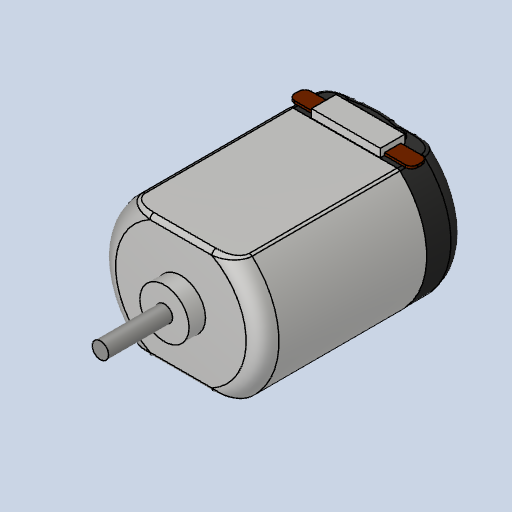
# Autodesk Inventor part: 3V DC Electromotor
Saved by Autodesk Inventor 2023 (Build 270158000, 158)
## iProperties
Created: 2020-10-25
Part Number: 3V DC Electromotor
Material: Aluminum 6061
Document SubType Name: Modeling
Designer: Niels
Density: 2.7 g/cm^3
Appearance: Aluminum - Flat
MAAT: ØLxBxD
Author: Niels
Autodesk Inventor part; units mm, degrees
ref_plane "YZ Plane" through (0, 0, 0) normal (1, 0, 0) x (0, 1, 0)
ref_plane "XZ Plane" through (0, 0, 0) normal (0, 1, 0) x (-1, 0, 0)
ref_plane "XY Plane" through (0, 0, 0) normal (0, 0, 1) x (1, 0, 0)
sketch "Sketch1" plane through (0, 0, 0) normal (0, 0, 1) x (1, 0, 0)
  circle A0 centre (0, 0) radius 9.95
  line L0 (-6.53854, 7.5) -> (6.53854, 7.5)
  line L1 (6.53854, -7.5) -> (-6.53854, -7.5)
  dimension "d0" = 19.9
  dimension "d2" = 15
  constraints: 4 end point, 4 point on circle, 1 centre point, 1 coincident, 1 horizontal, 1 parallel, 1 vertical alignment
  measures "d0" diameter of A0
  measures "d2" distance between parallel lines of L1 L0
extrude "Extrusion1" add sketch "Sketch1" along normal blind 20 contours A0 L1 L0
sketch "Sketch2" plane through (0, 0, 0) normal (0, 0, -1) x (-1, 0, 0)
  arc A0 (6.53854, -7.5) -> (6.53854, 7.5) centre (0, 0) ccw
  line L0 (-6.53854, 7.5) -> (6.53854, 7.5)
  arc A1 (-6.53854, 7.5) -> (-6.53854, -7.5) centre (0, 0) ccw
  line L1 (6.53854, -7.5) -> (-6.53854, -7.5)
  arc A2 (6.519778, -7.45) -> (6.519778, 7.45) centre (0, 0) ccw
  line L2 (6.519778, -7.45) -> (-6.519778, -7.45)
  arc A3 (-6.519778, 7.45) -> (-6.519778, -7.45) centre (0, 0) ccw
  line L3 (-6.519778, 7.45) -> (6.519778, 7.45)
  dimension "d5" = 0.05
  constraints: 4 end point, 4 point on circle, 2 centre point, 3 other
  measures "d5" distance between parallel lines of L0 L3
extrude "Extrusion2" add sketch "Sketch2" along normal blind 5 contours L2 A3 L3 A2
sketch "Sketch3" plane through (0, 0, 20) normal (0, 0, 1) x (1, 0, 0)
  circle A0 centre (0, 0) radius 3
  dimension "d8" = 6
  constraints: 1 centre point, 1 coincident
  measures "d8" diameter of A0
extrude "Extrusion3" add sketch "Sketch3" along normal blind 2
sketch "Sketch4" plane through (0, 0, 22) normal (0, 0, 1) x (1, 0, 0)
  circle A0 centre (0, 0) radius 1
  dimension "d11" = 2
  constraints: 1 centre point, 1 coincident
  measures "d11" diameter of A0
extrude "Extrusion4" add sketch "Sketch4" along normal blind 7.8
sketch "Sketch5" plane through (0, 0, -5) normal (0, 0, -1) x (-1, 0, 0)
  arc A0 (3.163068, -3.775) -> (-3.163068, -3.775) centre (0, 0) ccw
  line L0 (-3.163068, -3.775) -> (3.163068, -3.775)
  point P0 (0, 4.925)
  dimension "d14" = 9.85
  dimension "d15" = 8.7
  constraints: 3 point on circle, 2 end point, 1 centre point, 1 coincident, 1 horizontal, 1 vertical alignment
  measures "d14" diameter of A0
  measures "d15" distance from line of L0 point (0, 4.925)
extrude "Extrusion5" add sketch "Sketch5" along normal blind 2.2
sketch "Sketch6" plane through (0, 0, -7.2) normal (0, 0, -1) x (-1, 0, 0)
  circle A0 centre (0, 0) radius 1.8
  dimension "d18" = 3.6
  constraints: 1 centre point, 1 coincident
  measures "d18" diameter of A0
extrude "Extrusion6" cut sketch "Sketch6" against normal blind 0.1
sketch "Sketch7" plane through (0, 0, -7.1) normal (0, 0, -1) x (-1, 0, 0)
  circle A0 centre (0, 0) radius 1
  dimension "d21" = 2
  constraints: 1 centre point, 1 coincident
  measures "d21" diameter of A0
extrude "Extrusion7" add sketch "Sketch7" along normal blind 1
fillet "Fillet1" radius 0.5 4 edges at (3.1631, -3.775, -6.1) (-3.1631, -3.775, -6.1) (0, 4.925, -7.2) (0, -3.775, -7.2)
fillet "Fillet2" radius 2 4 edges at (-9.9, 0, -5) (9.9, 0, -5) (9.95, 0, 20) (-9.95, 0, 20)
fillet "Fillet3" radius 0.5 20 edges at (6.5385, 7.5, 9) (5.0788, 7.5, 19.6651) (0, 7.5, 20) (-5.0788, 7.5, 19.6651) (-6.5385, 7.5, 9) (5.0788, -7.5, 19.6651) (0, -7.5, 20) (-5.0788, -7.5, 19.6651) (-6.5385, -7.5, 9) (6.5385, -7.5, 9) (5.0647, -7.45, -4.6647) (0, -7.45, -5) (-5.0647, -7.45, -4.6647) (-6.5198, -7.45, -1.5) (6.5198, -7.45, -1.5) (5.0647, 7.45, -4.6647) (0, 7.45, -5) (-5.0647, 7.45, -4.6647) (-6.5198, 7.45, -1.5) (6.5198, 7.45, -1.5)
sketch "Sketch8" plane through (-6.329099, 7.45, 0) normal (0, 1, 0) x (1, 0, 0)
  line L0 (10.529099, 0.1) -> (2.129099, 0.1)
  line L1 (2.129099, 0.1) -> (2.129099, 3.1)
  line L2 (2.129099, 3.1) -> (10.529099, 3.1)
  line L3 (10.529099, 3.1) -> (10.529099, 0.1)
  line L4 (10.529099, 0.1) -> (2.129099, 3.1) construction
  line L5 (2.129099, 0.1) -> (10.529099, 3.1) construction
  line L6 (12.677524, 0) -> (-0.019326, 0)
  line L7 (2.604099, 3.11) -> (10.054099, 3.11)
  line L8 (10.054099, 3.11) -> (10.054099, 3.706558)
  line L9 (9.850005, 3.952307) -> (8.165305, 4.267003)
  line L10 (4.492894, 4.267003) -> (2.808194, 3.952307)
  line L11 (2.604099, 3.11) -> (2.604099, 3.706558)
  arc A0 (8.165305, 4.267003) -> (4.492894, 4.267003) centre (6.329099, -5.562969) ccw
  arc A1 (2.808194, 3.952307) -> (2.604099, 3.706558) centre (2.854099, 3.706558) ccw
  arc A2 (10.054099, 3.706558) -> (9.850005, 3.952307) centre (9.804099, 3.706558) ccw
  point P0 (6.329099, 0)
  point P1 (6.329099, 1.6)
  point P2 (6.329099, 1.6)
  point P3 (6.329099, 0)
  point P4 (10.054099, 3.914183)
  point P5 (6.329099, 4.61)
  point P6 (2.604099, 3.914183)
  point P7 (6.329099, 3.11)
  point P8 (6.329099, 1.6)
  dimension "d27" = 8.4
  dimension "d28" = 3
  dimension "d29" = 0.1
  dimension "d30" = 7.45
  dimension "d31" = 1.5
  dimension "d32" = 10
  dimension "d33" = 0.25
  dimension "d36" = 0.01
  constraints: 22 end point, 6 midpoint, 6 point on circle, 6 point on line, 6 tangent, 3 centre point, 3 vertical alignment, 2 horizontal, 2 parallel, 2 perpendicular, 1 equal radius, 1 horizontal alignment, 1 vertical
  measures "d27" distance of L1.end L2.end
  measures "d28" distance of L0.end L1.end
  measures "d29" distance from line of L0 point (6.329, 0)
  measures "d30" distance of L7.start L7.end
  measures "d31" distance from line of L7 point (6.329, 4.61)
  measures "d32" radius of A0
  measures "d33" radius of A1
  measures "d36" distance between parallel lines of L2 L7
extrude "Extrusion8" add sketch "Sketch8" along normal blind 1
sketch "Sketch9" plane through (-6.329099, 7.45, 0) normal (0, 1, 0) x (1, 0, 0)
  line L0 (-1.170901, 2.6) -> (13.829099, 2.6)
  line L1 (13.829099, 2.6) -> (13.829099, 0.6)
  line L2 (13.829099, 0.6) -> (-1.170901, 0.6)
  line L3 (-1.170901, 0.6) -> (-1.170901, 2.6)
  line L4 (2.129099, 0.1) -> (10.529099, 0.1)
  point P0 (6.329099, 0)
  point P1 (6.329099, 0.6)
  point P2 (6.329099, 0.1)
  dimension "d37" = 2
  dimension "d38" = 15
  dimension "d39" = 0.5
  constraints: 8 end point, 2 midpoint, 2 parallel, 1 horizontal, 1 perpendicular, 1 vertical alignment
  measures "d37" distance of L2.end L0.start
  measures "d38" distance of L0.start L0.end
  measures "d39" distance between parallel lines of L2 L4
extrude "Extrusion9" add sketch "Sketch9" along normal blind 0.3
fillet "Fillet4" radius 0.75 4 edges at (7.5, 7.6, -0.6) (7.5, 7.6, -2.6) (-7.5, 7.6, -0.6) (-7.5, 7.6, -2.6)
fillet "Fillet5" radius 0.75 7 edges at (0, 8.45, -4.437) (-2.6786, 8.45, -4.1097) (-3.6673, 8.45, -3.8663) (-3.725, 8.45, -3.4083) (2.6786, 8.45, -4.1097) (3.6673, 8.45, -3.8663) (3.725, 8.45, -3.4083)
body "Solid1"
